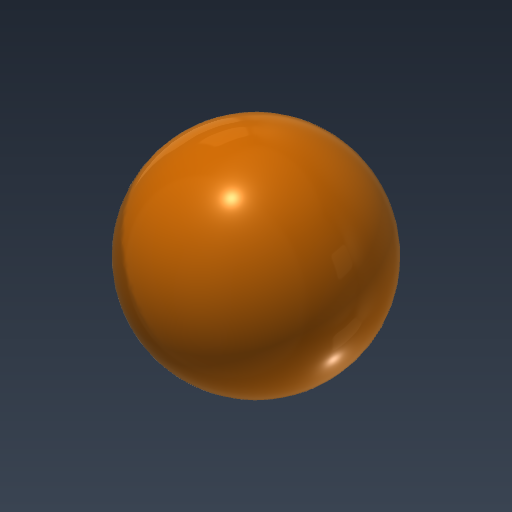
# Autodesk Inventor part: Golfball
Saved by Autodesk Inventor 2023.1 (Build 271208000, 208)
## iProperties
Created: 2012-07-15
Part Number: Golfball
Material: Golfball
Document SubType Name: Modeling
Designer: rYan
Mass: 44.1276 g
Surface Area: 58.088 cm^2
Volume: 41.6298 cm^3
Density: 1.06 g/cm^3
Appearance: Allgemein
Author: rYan
Autodesk Inventor part; units mm, degrees
ref_plane "YZ Plane" through (0, 0, 0) normal (1, 0, 0) x (0, 1, 0)
ref_plane "XZ Plane" through (0, 0, 0) normal (0, 1, 0) x (-1, 0, 0)
ref_plane "XY Plane" through (0, 0, 0) normal (0, 0, 1) x (1, 0, 0)
sketch "Skizze1" plane through (0, 0, 0) normal (0, 0, 1) x (1, 0, 0)
  circle A0 centre (0, 0) radius 21.5
  line L0 (-21.5, 0) -> (21.5, 0)
  line L1 (-30.1, 0) -> (30.1, 0) projected
  dimension "d0" = 43
  constraints: 2 end point, 2 point on circle, 1 centre point, 1 coincident, 1 collinear, 1 horizontal
  measures "d0" diameter of A0
revolve "Umdrehung1" add sketch "Skizze1" angle 360 about axis through (0, 0, 0) along (1, 0, 0) picked at (-4.2794, 7.6131) contours L0 A0
